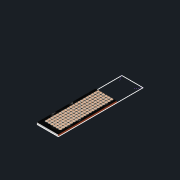
# Autodesk Inventor part: Proto-Board
Saved by Autodesk Inventor 2022.2 (Build 262287000, 287)
## iProperties
Created: 2022-02-20
Part Number: Proto-Board
Material: Generic
Document SubType Name: Modeling
Designer: Michael Lacey
Mass: 1.15891 g
Surface Area: 29.0097 cm^2
Volume: 1.15891 cm^3
Density: 1 g/cm^3
Appearance: Default
Author: Michael Lacey
Autodesk Inventor part; units mm, degrees
ref_plane "YZ Plane" through (0, 0, 0) normal (1, 0, 0) x (0, 1, 0)
ref_plane "XZ Plane" through (0, 0, 0) normal (0, 1, 0) x (-1, 0, 0)
ref_plane "XY Plane" through (0, 0, 0) normal (0, 0, 1) x (1, 0, 0)
sketch "Sketch1" plane through (0, 0, 0) normal (0, 1, 0) x (-1, 0, 0)
  line L0 (0, 0) -> (20, 0)
  line L1 (20, 0) -> (20, -80)
  line L2 (20, -80) -> (0, -80)
  line L3 (0, -80) -> (0, 0)
  circle A0 centre (3.65, -5.71) radius 1
  line L4 (3.65, -5.71) -> (0, 0) construction
  line L5 (16.35, -5.71) -> (20, 0) construction
  line L6 (16.35, -74.29) -> (20, -80) construction
  line L7 (3.65, -74.29) -> (0, -80) construction
  circle A1 centre (3.65, -5.71) radius 1.2835
  dimension "d0" = 20
  dimension "d1" = 80
  dimension "d2" = 2
  dimension "d32" = 5.71
  dimension "d33" = 3.65
  constraints: 16 end point, 2 centre point, 2 equal length, 2 parallel, 1 horizontal, 1 perpendicular
  measures "d0" distance of L1.end L2.end
  measures "d1" distance of L0.end L1.end
  measures "d2" diameter of A0
  measures "d32" distance from line of L0 L4.start
  measures "d33" distance from line of L3 L4.start
extrude "Extrusion1" add sketch "Sketch1" along normal blind 1.6 contours L0 L1 L2 L3 | A0 | A1
extrude "Extrusion4" cut sketch "Sketch1" along normal blind 1.6 contours A0
extrude "Extrusion5" cut sketch "Sketch1" along normal blind 0.01 contours A1
sketch "Sketch4" plane through (0, 1.6, 0) normal (0, 1, 0) x (1, 0, 0)
  circle A0 centre (-3.65, 5.71) radius 1 projected
  line L0 (0, 80) -> (-20, 80) projected
  line L1 (-20, 80) -> (-20, 0) projected
  line L2 (-20, 0) -> (0, 0) projected
  line L3 (0, 0) -> (0, 80) projected
  circle A1 centre (-3.65, 5.71) radius 1.397
  dimension "d38" = 2.794
  constraints: 1 centre point, 1 coincident
  measures "d38" diameter of A1
extrude "Extrusion6" cut sketch "Sketch4" against normal blind 0.01 contours A1
pattern_linear "Rectangular Pattern2" count 6 spacing 2.54 along (-1, 0, 0) count 20 spacing 2.54 along (0, 0, -1) of "Extrusion4", "Extrusion5", "Extrusion6"
sketch "Sketch5" plane through (0, 1.6, 0) normal (0, 1, 0) x (1, 0, 0)
  line L0 (0, 80) -> (-20, 80) projected
  line L1 (-20, 80) -> (-20, 0) projected
  line L2 (-20, 0) -> (0, 0) projected
  line L3 (0, 0) -> (0, 80) projected
  arc A0 (-7.46, 5.128) -> (-4.92, 5.128) centre (-6.19, 5.71) ccw projected
  arc A1 (-10, 5.128) -> (-7.46, 5.128) centre (-8.73, 5.71) ccw projected
  arc A2 (-12.54, 5.128) -> (-10, 5.128) centre (-11.27, 5.71) ccw projected
  arc A3 (-15.08, 5.128) -> (-12.54, 5.128) centre (-13.81, 5.71) ccw projected
  arc A4 (-16.932, 6.98) -> (-15.08, 5.128) centre (-16.35, 5.71) ccw projected
  arc A5 (-16.932, 9.52) -> (-16.932, 6.98) centre (-16.35, 8.25) ccw projected
  arc A6 (-16.932, 12.06) -> (-16.932, 9.52) centre (-16.35, 10.79) ccw projected
  arc A7 (-16.932, 14.6) -> (-16.932, 12.06) centre (-16.35, 13.33) ccw projected
  arc A8 (-16.932, 17.14) -> (-16.932, 14.6) centre (-16.35, 15.87) ccw projected
  arc A9 (-16.932, 19.68) -> (-16.932, 17.14) centre (-16.35, 18.41) ccw projected
  arc A10 (-16.932, 22.22) -> (-16.932, 19.68) centre (-16.35, 20.95) ccw projected
  arc A11 (-16.932, 24.76) -> (-16.932, 22.22) centre (-16.35, 23.49) ccw projected
  arc A12 (-16.932, 27.3) -> (-16.932, 24.76) centre (-16.35, 26.03) ccw projected
  arc A13 (-16.932, 29.84) -> (-16.932, 27.3) centre (-16.35, 28.57) ccw projected
  arc A14 (-16.932, 32.38) -> (-16.932, 29.84) centre (-16.35, 31.11) ccw projected
  arc A15 (-16.932, 34.92) -> (-16.932, 32.38) centre (-16.35, 33.65) ccw projected
  arc A16 (-16.932, 37.46) -> (-16.932, 34.92) centre (-16.35, 36.19) ccw projected
  arc A17 (-16.932, 40) -> (-16.932, 37.46) centre (-16.35, 38.73) ccw projected
  arc A18 (-16.932, 42.54) -> (-16.932, 40) centre (-16.35, 41.27) ccw projected
  arc A19 (-16.932, 45.08) -> (-16.932, 42.54) centre (-16.35, 43.81) ccw projected
  arc A20 (-16.932, 47.62) -> (-16.932, 45.08) centre (-16.35, 46.35) ccw projected
  arc A21 (-16.932, 50.16) -> (-16.932, 47.62) centre (-16.35, 48.89) ccw projected
  arc A22 (-16.932, 52.7) -> (-16.932, 50.16) centre (-16.35, 51.43) ccw projected
  arc A23 (-15.768, 52.7) -> (-15.08, 53.388) centre (-16.35, 53.97) ccw projected
  arc A24 (-4.92, 53.388) -> (-4.232, 52.7) centre (-3.65, 53.97) ccw projected
  arc A25 (-3.068, 50.16) -> (-3.068, 52.7) centre (-3.65, 51.43) ccw projected
  arc A26 (-3.068, 47.62) -> (-3.068, 50.16) centre (-3.65, 48.89) ccw projected
  arc A27 (-3.068, 45.08) -> (-3.068, 47.62) centre (-3.65, 46.35) ccw projected
  arc A28 (-3.068, 42.54) -> (-3.068, 45.08) centre (-3.65, 43.81) ccw projected
  arc A29 (-3.068, 40) -> (-3.068, 42.54) centre (-3.65, 41.27) ccw projected
  arc A30 (-3.068, 37.46) -> (-3.068, 40) centre (-3.65, 38.73) ccw projected
  arc A31 (-3.068, 34.92) -> (-3.068, 37.46) centre (-3.65, 36.19) ccw projected
  arc A32 (-3.068, 32.38) -> (-3.068, 34.92) centre (-3.65, 33.65) ccw projected
  arc A33 (-3.068, 29.84) -> (-3.068, 32.38) centre (-3.65, 31.11) ccw projected
  arc A34 (-3.068, 27.3) -> (-3.068, 29.84) centre (-3.65, 28.57) ccw projected
  arc A35 (-3.068, 24.76) -> (-3.068, 27.3) centre (-3.65, 26.03) ccw projected
  arc A36 (-3.068, 22.22) -> (-3.068, 24.76) centre (-3.65, 23.49) ccw projected
  arc A37 (-3.068, 19.68) -> (-3.068, 22.22) centre (-3.65, 20.95) ccw projected
  arc A38 (-3.068, 17.14) -> (-3.068, 19.68) centre (-3.65, 18.41) ccw projected
  arc A39 (-3.068, 14.6) -> (-3.068, 17.14) centre (-3.65, 15.87) ccw projected
  arc A40 (-3.068, 12.06) -> (-3.068, 14.6) centre (-3.65, 13.33) ccw projected
  arc A41 (-3.068, 9.52) -> (-3.068, 12.06) centre (-3.65, 10.79) ccw projected
  arc A42 (-3.068, 6.98) -> (-3.068, 9.52) centre (-3.65, 8.25) ccw projected
  arc A43 (-4.92, 5.128) -> (-3.068, 6.98) centre (-3.65, 5.71) ccw projected
  line L4 (0, 80) -> (-20, 80)
  line L5 (-20, 80) -> (-20, 55.24)
  line L6 (-20, 55.24) -> (0, 55.24)
  line L7 (0, 55.24) -> (0, 80)
  arc A44 (-15.08, 52.012) -> (-15.768, 52.7) centre (-16.35, 51.43) ccw projected
  arc A45 (-14.392, 52.7) -> (-15.08, 52.012) centre (-13.81, 51.43) ccw projected
  arc A46 (-15.08, 53.388) -> (-14.392, 52.7) centre (-13.81, 53.97) ccw projected
  arc A47 (-15.08, 54.552) -> (-16.932, 52.7) centre (-16.35, 53.97) ccw projected
  arc A48 (-12.54, 54.552) -> (-15.08, 54.552) centre (-13.81, 53.97) ccw projected
  arc A49 (-10, 54.552) -> (-12.54, 54.552) centre (-11.27, 53.97) ccw projected
  arc A50 (-7.46, 54.552) -> (-10, 54.552) centre (-8.73, 53.97) ccw projected
  arc A51 (-4.92, 54.552) -> (-7.46, 54.552) centre (-6.19, 53.97) ccw projected
  arc A52 (-3.068, 52.7) -> (-4.92, 54.552) centre (-3.65, 53.97) ccw projected
  arc A53 (-5.608, 52.7) -> (-4.92, 53.388) centre (-6.19, 53.97) ccw projected
  arc A54 (-4.92, 52.012) -> (-5.608, 52.7) centre (-6.19, 51.43) ccw projected
  arc A55 (-4.232, 52.7) -> (-4.92, 52.012) centre (-3.65, 51.43) ccw projected
  constraints: 8 end point, 2 parallel, 1 horizontal, 1 perpendicular, 1 point on line
extrude "Extrusion7" cut sketch "Sketch5" against normal blind 25.4 contours L3 L6 A52 A51 A50 A49 A48 A47 L1 L0 | L6 A52 | A47 L6 | L6 A51 | A48 L6 | L6 A50 | A49 L6
body "Solid1"
